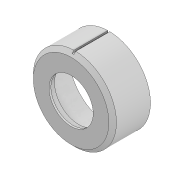
# Autodesk Inventor part: PolarizerObjectiveCap-MitutoyoPlanApoBD
Saved by Autodesk Inventor 2021 (Build 250183000, 183)
## iProperties
Created: 2023-02-07
Part Number: PolarizerObjectiveCap-MitutoyoPlanApoBD
Material: Generic
Document SubType Name: Modeling
Designer: nvladi
Density: 1 g/cm^3
Appearance: Default
Author: nvladi
Autodesk Inventor part; units mm, degrees
ref_plane "YZ Plane" through (0, 0, 0) normal (1, 0, 0) x (0, 1, 0)
ref_plane "XZ Plane" through (0, 0, 0) normal (0, 1, 0) x (-1, 0, 0)
ref_plane "XY Plane" through (0, 0, 0) normal (0, 0, 1) x (1, 0, 0)
sketch "Sketch1" plane through (0, 0, 0) normal (0, 0, 1) x (1, 0, 0)
  circle A0 centre (0, 0) radius 21.1
  circle A1 centre (0, 0) radius 22
  circle A2 centre (0, 0) radius 12.8
  circle A3 centre (0, 0) radius 11.7
  circle A4 centre (0, 22) radius 0.5
  dimension "d1" = 44
  dimension "d0" = 42.2
  dimension "d2" = 25.6
  dimension "d3" = 23.4
  dimension "d13" = 1
  constraints: 4 centre point, 4 coincident, 1 vertical alignment, 2 other
  measures "d0" diameter of A0
  measures "d2" diameter of A2
  measures "d3" diameter of A3
  measures "d13" diameter of A4
extrude "Extrusion1" add sketch "Sketch1" against normal blind 4 contours A0
extrude "Extrusion2" add sketch "Sketch1" against normal blind 20 contours A1 A4 | A4 A1 picked at (5.1126, 20.6747) picked at (0.0199, 21.8341)
extrude "Extrusion3" add sketch "Sketch1" against normal blind 1 contours A2
chamfer "Chamfer1" distance 2 angle 45 1 edges at (-22, 0, 0)
sketch "Sketch2" plane through (0, 0, -20) normal (0, 0, -1) x (-1, 0, 0)
  circle A0 centre (0, 0) radius 22 projected
  line L0 (0.5, 21) -> (-0.5, 21)
  line L1 (-0.5, 21) -> (-0.5, 23)
  line L2 (-0.5, 23) -> (0.5, 23)
  line L3 (0.5, 23) -> (0.5, 21)
  line L4 (0.5, 21) -> (-0.5, 23) construction
  line L5 (-0.5, 21) -> (0.5, 23) construction
  point P0 (0, 22)
  dimension "d15" = 1
  dimension "d16" = 2
  constraints: 12 end point, 2 midpoint, 2 parallel, 1 horizontal, 1 perpendicular, 1 vertical alignment, 1 other
  measures "d15" distance of L1.end L2.end
  measures "d16" distance of L0.end L1.end
extrude "Extrusion4" cut sketch "Sketch2" against normal blind 20 contours L3 L0 L1 A0 | A0 L1 L2 L3 picked at (-0.0556, 21.3331)
body "Solid1"
